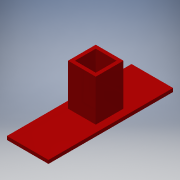
# Autodesk Inventor part: mounting plate
Saved by Autodesk Inventor 2016 (Build 200138000, 138)
## iProperties
Created: 2016-01-17
Part Number: mounting plate
Material: ABS Plastic
Document SubType Name: Modeling
Designer: gus
Density: 1.06 g/cm^3
Appearance: Smooth - Red
Mass: 25.9872 g
Surface Area: 164.617 cm^2
Volume: 24.5162 cm^3
Author: gus
Autodesk Inventor part; units mm, degrees
ref_plane "YZ Plane" through (0, 0, 0) normal (1, 0, 0) x (0, 1, 0)
ref_plane "XZ Plane" through (0, 0, 0) normal (0, 1, 0) x (-1, 0, 0)
ref_plane "XY Plane" through (0, 0, 0) normal (0, 0, 1) x (1, 0, 0)
sketch "Sketch1" plane through (0, 0, 0) normal (0, 1, 0) x (-1, 0, 0)
  line L0 (0, 0) -> (-38.1, 0)
  line L1 (-38.1, 0) -> (-38.1, -114.3)
  line L2 (-38.1, -114.3) -> (0, -114.3)
  line L3 (0, -114.3) -> (0, 0)
  dimension "d0" = 38.1
  dimension "d1" = 114.3
  constraints: 8 end point, 2 parallel, 1 horizontal, 1 perpendicular
  measures "d0" distance of L2.end L1.end
  measures "d1" distance of L1.end L0.end
extrude "Extrusion1" add sketch "Sketch1" along normal blind 3.175
sketch "Sketch3" plane through (0, 3.175, 0) normal (0, 1, 0) x (1, 0, 0)
  line L0 (31.75, 62.4332) -> (6.35, 62.4332)
  line L1 (6.35, 62.4332) -> (6.35, 37.0332)
  line L2 (6.35, 37.0332) -> (31.75, 37.0332)
  line L3 (31.75, 37.0332) -> (31.75, 62.4332)
  line L4 (38.1, 0) -> (38.1, 114.3) projected
  line L5 (38.1, 114.3) -> (0, 114.3) projected
  line L6 (28.575, 59.2582) -> (9.525, 59.2582)
  line L7 (9.525, 59.2582) -> (9.525, 40.2082)
  line L8 (9.525, 40.2082) -> (28.575, 40.2082)
  line L9 (28.575, 40.2082) -> (28.575, 59.2582)
  circle A0 centre (19.05, 49.7332) radius 2.54
  line L10 (0, 0) -> (38.1, 0) projected
  dimension "d8" = 25.4
  dimension "d9" = 25.4
  dimension "d10" = 6.35
  dimension "d12" = 3.175
  dimension "d15" = 5.08
  dimension "d16" = 12.7
  dimension "d17" = 12.7
  dimension "d23" = 37.0332
  constraints: 16 end point, 4 parallel, 2 perpendicular, 1 centre point, 1 horizontal, 3 other
  measures "d8" distance of L2.end L1.end
  measures "d9" distance of L1.end L0.end
  measures "d10" distance between parallel lines of L4 L3
  measures "d12" distance between parallel lines of L3 L9
  measures "d15" diameter of A0
  measures "d16" distance from line of L1 A0.centre
  measures "d17" distance from line of L2 A0.centre
  measures "d23" distance between parallel lines of L10 L2
extrude "Extrusion3" add sketch "Sketch3" along normal blind 38.1 contours L3 L2 L1 L0
extrude "Extrusion5" cut sketch "Sketch3" against normal blind 3.175 contours A0
body "Solid1"
